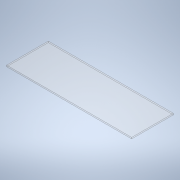
# Autodesk Inventor part: new topsides
Saved by Autodesk Inventor 2020.1 (Build 241239000, 239)
## iProperties
Created: 2021-08-04
Part Number: new topsides
Material: PMMA Plastic
Document SubType Name: Modeling
Designer: Caleb
Density: 1.188 g/cm^3
Appearance: Polycarbonate - Clear
Author: Caleb
Autodesk Inventor part; units mm, degrees
ref_plane "YZ Plane" through (0, 0, 0) normal (1, 0, 0) x (0, 1, 0)
ref_plane "XZ Plane" through (0, 0, 0) normal (0, 1, 0) x (-1, 0, 0)
ref_plane "XY Plane" through (0, 0, 0) normal (0, 0, 1) x (1, 0, 0)
sketch "Sketch1" plane through (0, 0, 0) normal (0, 1, 0) x (-1, 0, 0)
  line L0 (-225, 76.6304) -> (225, 76.6304)
  line L1 (225, 76.6304) -> (225, -73.3696)
  line L2 (225, -73.3696) -> (-225, -73.3696)
  line L3 (-225, -73.3696) -> (-225, 76.6304)
  point P0 (0, 0)
  dimension "d4" = 450
  dimension "d5" = 150
  constraints: 8 end point, 2 parallel, 1 horizontal, 1 perpendicular
  measures "d4" distance between parallel lines of L1 L3
  measures "d5" distance of L0.end L1.end
extrude "Extrusion1" add sketch "Sketch1" along normal mid plane 5
body "Solid1"
